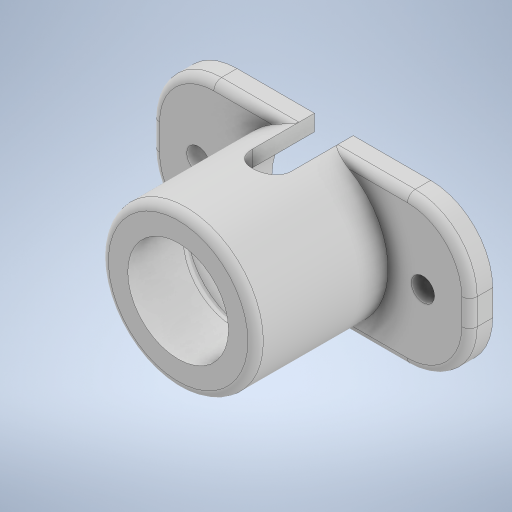
# Autodesk Inventor part: cover.ver1
Saved by Autodesk Inventor 2023 (Build 270158000, 158)
## iProperties
Created: 2023-11-07
Part Number: cover.ver1
Material: 一般
Document SubType Name: Modeling
Designer: bonju
Density: 1 g/cm^3
Appearance: 既定
Author: bonju
Autodesk Inventor part; units mm, degrees
ref_plane "YZ Plane" through (0, 0, 0) normal (1, 0, 0) x (0, 1, 0)
ref_plane "XZ Plane" through (0, 0, 0) normal (0, 1, 0) x (-1, 0, 0)
ref_plane "XY Plane" through (0, 0, 0) normal (0, 0, 1) x (1, 0, 0)
sketch "スケッチ1" plane through (0, 0, 0) normal (0, 0, 1) x (1, 0, 0)
  circle A0 centre (0, 0) radius 8
  circle A1 centre (0, 0) radius 10
  dimension "d0" = 16
  dimension "d1" = 2
  constraints: 2 centre point, 1 coincident
  measures "d0" diameter of A0
  measures "d1" radial gap between concentric circles of A0 A1
extrude "押し出し1" add sketch "スケッチ1" along normal blind 12
sketch "スケッチ2" plane through (0, 0, 12) normal (0, 0, 1) x (1, 0, 0)
  circle A0 centre (0, 0) radius 6.5
  circle A1 centre (0, 0) radius 10 projected
  circle A2 centre (0, 0) radius 10
  dimension "d4" = 13
  constraints: 2 centre point, 2 coincident
  measures "d4" diameter of A0
extrude "押し出し2" add sketch "スケッチ2" along normal blind 8.1
sketch "スケッチ3" plane through (0, 0, 0) normal (0, 1, 0) x (-1, 0, 0)
  line L0 (10, 0) -> (-10, 0) projected
  line L1 (2.5, 0) -> (2.5, 8)
  arc A0 (2.5, 8) -> (-2.5, 8) centre (0, 8) ccw
  line L2 (-2.5, 8) -> (-2.5, 0)
  line L3 (2.5, 0) -> (-2.5, 0)
  line L4 (0, -2.1) -> (0, 12.6) projected
  point P0 (0, 0)
  dimension "d7" = 5
  dimension "d8" = 8
  constraints: 6 end point, 2 point on circle, 2 point on line, 2 tangent, 1 centre point, 1 collinear, 1 parallel, 1 vertical, 1 other
  measures "d7" distance between parallel lines of L2 L1
  measures "d8" distance of L1.start L1.end
extrude "押し出し3" cut sketch "スケッチ3" along normal through all both and the other way through all
fillet "フィレット1" radius 1 2 edges at (-8, 0, 12) (-6.5, 0, 12)
fillet "フィレット2" radius 1 1 edges at (-10, 0, 20.1)
sketch "スケッチ4" plane through (0, 0, 0) normal (0, 0, -1) x (-1, 0, 0)
  line L0 (2.5, -9.6825) -> (2.5, -7.5993) projected
  line L1 (2.5, -9.6825) -> (20.5, -9.6825)
  circle A0 centre (0, 0) radius 10 projected
  line L2 (2.5, 9.6825) -> (20.5, 9.6825)
  line L3 (20.5, 9.6825) -> (20.5, -9.6825)
  line L4 (2.5, 7.5993) -> (2.5, 9.6825) projected
  arc A1 (2.5, -9.6825) -> (2.5, 9.6825) centre (0, 0) ccw
  line L5 (0, -14) -> (0, 14) projected
  line L6 (-2.5, -9.6825) -> (-20.5, -9.6825)
  line L7 (-2.5, 9.6825) -> (-20.5, 9.6825)
  line L8 (-20.5, 9.6825) -> (-20.5, -9.6825)
  arc A2 (-2.5, 9.6825) -> (-2.5, -9.6825) centre (0, 0) ccw
  point P0 (-2.5, -9.6825)
  dimension "d13" = 18
  constraints: 12 end point, 5 point on circle, 4 symmetric about line, 2 centre point, 2 horizontal, 1 coincident, 1 perpendicular, 1 other
  measures "d13" distance of L0.start L1.end
extrude "押し出し4" add sketch "スケッチ4" against normal blind 3 contours A0 L2 L3 L1 | L6 L8 L7 A0
fillet "フィレット3" radius 8 4 edges at (20.5, 9.6825, 1.5) (20.5, -9.6825, 1.5) (-20.5, -9.6825, 1.5) (-20.5, 9.6825, 1.5)
fillet "フィレット4" radius 1 10 edges at (-18.1569, -7.3393, 3) (-7.5, -9.6825, 3) (-18.1569, 7.3393, 3) (-7.5, 9.6825, 3) (-20.5, 0, 3) (18.1569, 7.3393, 3) (7.5, 9.6825, 3) (18.1569, -7.3393, 3) (7.5, -9.6825, 3) (20.5, 0, 3)
sketch "スケッチ5" plane through (0, 0, 3) normal (0, 0, 1) x (1, 0, 0)
  circle A0 centre (14.5, 0) radius 1.5
  circle A1 centre (0, 0) radius 10 projected
  line L0 (-28.7, 0) -> (28.7, 0) projected
  line L1 (0, -14.0024) -> (0, 14.0024) projected
  circle A2 centre (-14.5, 0) radius 1.5
  dimension "d18" = 3
  dimension "d19" = 3
  constraints: 2 centre point, 1 point on line, 1 symmetric about line, 1 other
  measures "d18" diameter of A0
extrude "押し出し5" cut sketch "スケッチ5" against normal through all contours L0 A0 | A0 L0 | A2 L0 | L0 A2
